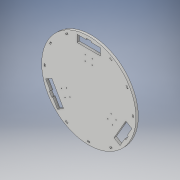
# Autodesk Inventor part: denew
Saved by Autodesk Inventor 2019 (Build 230136000, 136)
## iProperties
Created: 2021-01-20
Part Number: denew
Material: Generic
Document SubType Name: Modeling
Designer: Admin
Density: 1 g/cm^3
Appearance: Default
Author: Admin
Autodesk Inventor part; units mm, degrees
ref_plane "YZ Plane" through (0, 0, 0) normal (1, 0, 0) x (0, 1, 0)
ref_plane "XZ Plane" through (0, 0, 0) normal (0, 1, 0) x (-1, 0, 0)
ref_plane "XY Plane" through (0, 0, 0) normal (0, 0, 1) x (1, 0, 0)
sketch "Sketch1" plane through (0, 0, 0) normal (0, 0, 1) x (1, 0, 0)
  circle A0 centre (0, 0) radius 200
  line L0 (90.6699, 167.0448) -> (88.1699, 162.7147)
  line L1 (96.8301, 157.7147) -> (99.3301, 162.0448)
  line L2 (162.0448, 99.3301) -> (157.7147, 96.8301)
  line L3 (162.7147, 88.1699) -> (167.0448, 90.6699)
  line L4 (185, 5) -> (190, 5)
  line L5 (190, -5) -> (185, -5)
  line L6 (88.1699, -162.7147) -> (96.8301, -157.7147)
  line L7 (99.3301, -162.0448) -> (90.6699, -167.0448)
  line L8 (-5, -190) -> (-5, -185)
  line L9 (5, -185) -> (5, -190)
  line L10 (-99.3301, -162.0448) -> (-90.6699, -167.0448)
  line L11 (-88.1699, -162.7147) -> (-96.8301, -157.7147)
  line L12 (-190, 5) -> (-190, -5)
  line L13 (-190, -5) -> (-185, -5)
  line L14 (-185, -5) -> (-185, 5)
  line L15 (-167.0448, 90.6699) -> (-162.0448, 99.3301)
  line L16 (-157.7147, 96.8301) -> (-162.7147, 88.1699)
  line L17 (-99.3301, 162.0448) -> (-90.6699, 167.0448)
  line L18 (-88.1699, 162.7147) -> (-96.8301, 157.7147)
  line L19 (-190, -5) -> (-190, 5)
  line L20 (-185, 5) -> (-185, -5)
  line L21 (88.1699, 162.7147) -> (96.8301, 157.7147)
  line L22 (99.3301, 162.0448) -> (90.6699, 167.0448)
  line L23 (162.7147, 88.1699) -> (157.7147, 96.8301)
  line L24 (162.0448, 99.3301) -> (167.0448, 90.6699)
  line L25 (185, 5) -> (185, -5)
  line L26 (190, 5) -> (190, -5)
  line L27 (96.8301, -157.7147) -> (99.3301, -162.0448)
  line L28 (88.1699, -162.7147) -> (90.6699, -167.0448)
  line L29 (-5, -185) -> (5, -185)
  line L30 (-5, -190) -> (5, -190)
  line L31 (-99.3301, -162.0448) -> (-96.8301, -157.7147)
  line L32 (-90.6699, -167.0448) -> (-88.1699, -162.7147)
  line L33 (-190, 5) -> (-185, 5)
  line L34 (-162.0448, 99.3301) -> (-157.7147, 96.8301)
  line L35 (-167.0448, 90.6699) -> (-162.7147, 88.1699)
  line L36 (-99.3301, 162.0448) -> (-96.8301, 157.7147)
  line L37 (-90.6699, 167.0448) -> (-88.1699, 162.7147)
  line L38 (50, 182.5) -> (10, 182.5)
  line L39 (10, 182.5) -> (10, 187.5)
  line L40 (10, 187.5) -> (0, 187.5)
  line L41 (157.7147, 96.8301) -> (162.0448, 99.3301)
  line L42 (167.0448, 90.6699) -> (162.7147, 88.1699)
  line L43 (-99.3301, -162.0448) -> (-96.8301, -157.7147)
  line L44 (-88.1699, -162.7147) -> (-90.6699, -167.0448)
  line L45 (-99.3301, -162.0448) -> (-96.8301, -157.7147)
  line L46 (-88.1699, -162.7147) -> (-90.6699, -167.0448)
  line L47 (-99.3301, -162.0448) -> (-90.6699, -167.0448)
  circle A1 centre (14.945, 125) radius 1.73
  circle A2 centre (14.945, 100.94) radius 1.73
  circle A3 centre (-14.945, 100.94) radius 1.73
  circle A4 centre (-14.945, 125) radius 1.73
  circle A5 centre (-100.7807, -75.4427) radius 1.73
  circle A6 centre (-115.7257, -49.5573) radius 1.73
  circle A7 centre (-79.9441, -63.4127) radius 1.73
  circle A8 centre (-94.8891, -37.5273) radius 1.73
  circle A9 centre (115.7257, -49.5573) radius 1.73
  circle A10 centre (100.7807, -75.4427) radius 1.73
  circle A11 centre (94.8891, -37.5273) radius 1.73
  circle A12 centre (79.9441, -63.4127) radius 1.73
  line L48 (0, 152.5) -> (50, 152.5)
  line L49 (50, 152.5) -> (50, 182.5)
  line L50 (-10, 182.5) -> (-10, 187.5)
  line L51 (-10, 187.5) -> (0, 187.5)
  line L52 (-50, 182.5) -> (-10, 182.5)
  line L53 (0, 152.5) -> (-50, 152.5)
  line L54 (-50, 152.5) -> (-50, 182.5)
  circle A13 centre (0, 0) radius 200
  line L55 (-163.0496, -82.5897) -> (-167.3798, -85.0897)
  line L56 (-167.3798, -85.0897) -> (-162.3798, -93.75)
  line L57 (-183.0496, -47.9487) -> (-163.0496, -82.5897)
  line L58 (-132.0689, -76.25) -> (-157.0689, -32.9487)
  line L59 (-157.0689, -32.9487) -> (-183.0496, -47.9487)
  line L60 (-132.0689, -76.25) -> (-107.0689, -119.5513)
  line L61 (-157.3798, -102.4103) -> (-162.3798, -93.75)
  line L62 (-153.0496, -99.9103) -> (-157.3798, -102.4103)
  line L63 (-133.0496, -134.5513) -> (-153.0496, -99.9103)
  line L64 (-107.0689, -119.5513) -> (-133.0496, -134.5513)
  circle A14 centre (0, 0) radius 200
  line L65 (153.0496, -99.9103) -> (157.3798, -102.4103)
  line L66 (157.3798, -102.4103) -> (162.3798, -93.75)
  line L67 (133.0496, -134.5513) -> (153.0496, -99.9103)
  line L68 (132.0689, -76.25) -> (107.0689, -119.5513)
  line L69 (107.0689, -119.5513) -> (133.0496, -134.5513)
  line L70 (132.0689, -76.25) -> (157.0689, -32.9487)
  line L71 (167.3798, -85.0897) -> (162.3798, -93.75)
  line L72 (163.0496, -82.5897) -> (167.3798, -85.0897)
  line L73 (183.0496, -47.9487) -> (163.0496, -82.5897)
  line L74 (157.0689, -32.9487) -> (183.0496, -47.9487)
  dimension "d6" = 40
  dimension "d8" = 3.46
  dimension "d9" = 360
  dimension "d11" = 50
  dimension "d14" = 360
  constraints: 150 end point, 15 centre point, 11 equal length, 9 perpendicular, 3 vertical, 2 coincident, 2 horizontal, 2 point on line, 90 other
  measures "d6" distance of L38.start L39.start
  measures "d8" diameter of A1
  measures "d11" distance of L48.start L48.end
extrude "Extrusion1" add sketch "Sketch1" along normal blind 10
body "Solid1"
